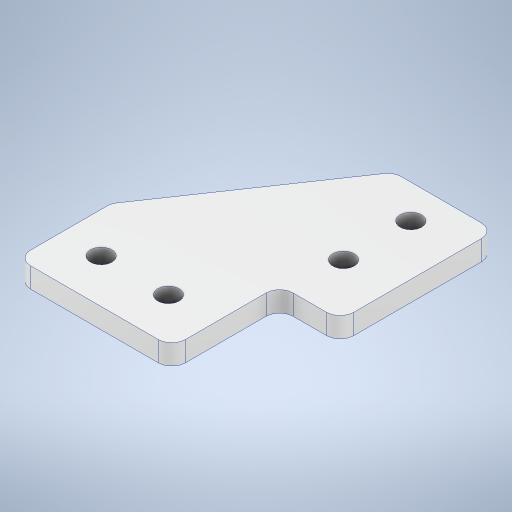
# Autodesk Inventor part: 射出_固定4
Saved by Autodesk Inventor 2023 (Build 270158000, 158)
## iProperties
Created: 2022-04-21
Part Number: 射出_固定4
Material: アルミニウム 6061
Document SubType Name: Modeling
Designer: yuta
Density: 2.7 g/cm^3
Appearance: アルミニウム - フラット
Author: yuta
Autodesk Inventor part; units mm, degrees
ref_plane "YZ Plane" through (0, 0, 0) normal (1, 0, 0) x (0, 1, 0)
ref_plane "XZ Plane" through (0, 0, 0) normal (0, 1, 0) x (-1, 0, 0)
ref_plane "XY Plane" through (0, 0, 0) normal (0, 0, 1) x (1, 0, 0)
sketch "スケッチ1" plane through (0, 0, 0) normal (0, 1, 0) x (-1, 0, 0)
  line L0 (40, 0) -> (40, -15)
  line L1 (40, -40) -> (23, -40) construction
  line L2 (0, -40) -> (0, 0)
  line L3 (40, -1) -> (0, -1)
  line L4 (40, -15) -> (23, -40)
  line L5 (8, -17) -> (0, -17)
  line L6 (8, -17) -> (8, -40) construction
  line L7 (17, -1) -> (17, -17)
  line L8 (17, -17) -> (8, -17)
  line L9 (23, -40) -> (0, -40)
  line L10 (40, -15) -> (40, -40) construction
  point P0 (17, 0)
  dimension "d0" = 40
  dimension "d1" = 40
  dimension "d2" = 17
  dimension "d3" = 8
  dimension "d4" = 15
  dimension "d5" = 15
  dimension "d7" = 17
  constraints: 22 end point, 7 point on line, 3 parallel, 3 perpendicular, 1 coincident, 1 horizontal
  measures "d0" distance of L1.start L2.start
  measures "d1" distance of L0.start L1.start
  measures "d2" distance of L2.end point (17, 0)
  measures "d3" distance of L2.start L6.end
  measures "d4" distance of L6.end L1.end
  measures "d5" distance of L0.start L0.end
  measures "d7" distance of L2.end L5.end
extrude "押し出し1" add sketch "スケッチ1" along normal blind 3 contours L0 L4 L9 L2 L5 L8 L7 L3
sketch "スケッチ2" plane through (0, 3, 0) normal (0, 1, 0) x (1, 0, 0)
  line L0 (0, 0) -> (-40, 0) construction
  line L1 (-40, 0) -> (-40, 40) construction
  line L2 (-40, 40) -> (0, 40) construction
  line L3 (0, 40) -> (0, 0) construction
  line L4 (-40, 15) -> (-40, 1) projected
  line L5 (-40, 15) -> (0, 15) construction
  line L6 (-23, 0) -> (-23, 43.077) construction
  line L7 (-40, 1) -> (-17, 1) projected
  point P0 (-34, 7.5)
  point P1 (-24, 7.5)
  point P2 (-15.5, 25)
  point P3 (-15.5, 35)
  dimension "d28" = 118
  dimension "d10" = 40
  dimension "d11" = 40
  dimension "d12" = 15
  dimension "d13" = 23
  dimension "d14" = 34
  dimension "d15" = 6.5
  dimension "d16" = 10
  dimension "d17" = 7.5
  dimension "d18" = 25
  dimension "d19" = 7.5
  dimension "d20" = 10
  dimension "d21" = 7.5
  constraints: 12 end point, 3 point on line, 2 parallel, 2 perpendicular, 1 horizontal, 1 vertical
  measures "d10" distance of L1.end L2.end
  measures "d11" distance of L0.end L1.end
  measures "d12" distance from line of L0.start L5
  measures "d13" distance between parallel lines of L3 L6
  measures "d14" distance from line of L3 point (-34, 7.5)
  measures "d15" distance from line of L7 point (-34, 7.5)
  measures "d16" distance of point (-34, 7.5) point (-24, 7.5)
  measures "d17" distance from line of L0 point (-24, 7.5)
  measures "d18" distance from line of point (-15.5, 25) L0
  measures "d19" distance from line of L6 point (-15.5, 25)
  measures "d20" distance of point (-15.5, 25) point (-15.5, 35)
  measures "d21" distance from line of L6 point (-15.5, 35)
hole "穴1" at (-34, 3, -7.5) at (-24, 3, -7.5) at (-15.5, 3, -25) at (-15.5, 3, -35) direction (0, -1, 0) diameter 3.2 end through all
sketch "スケッチ3" plane through (0, 3, 0) normal (0, 1, 0) x (1, 0, 0)
  line L0 (-17, 17) -> (0, 17) projected
  line L1 (0, 40) -> (-23, 40) projected
  line L2 (0, 17) -> (-8, 17)
  line L3 (-8, 17) -> (-8, 40)
  line L4 (-8, 40) -> (0, 40)
  line L5 (0, 40) -> (0, 17)
  point P0 (0, 0)
  dimension "d29" = 8
  dimension "d30" = 23
  constraints: 8 end point, 2 parallel, 1 horizontal, 1 perpendicular
  measures "d29" distance of L3.end L4.end
  measures "d30" distance of L2.end L3.end
extrude "押し出し2" cut sketch "スケッチ3" against normal blind 3
fillet "フィレット1" radius 2 7 edges at (-23, 1.5, -40) (-40, 1.5, -15) (-40, 1.5, -1) (-8, 1.5, -40) (-8, 1.5, -17) (-17, 1.5, -17) (-17, 1.5, -1)
